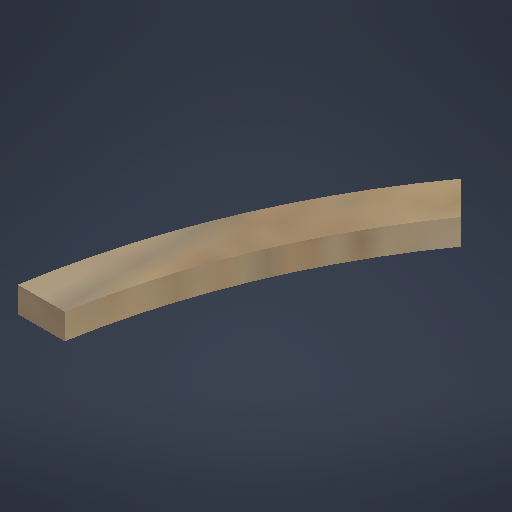
# Autodesk Inventor part: back_upper
Saved by Autodesk Inventor 2026.1 (Build 301233020, 233B)
## iProperties
Created: 2025-09-27
Part Number: back_upper
Material: 木材 (カエデ材)
Document SubType Name: Modeling
Designer: hibik
Density: 0.67 g/cm^3
Appearance: ナチュラル カエデ材 - 光沢 濃い着色
Author: hibik
Autodesk Inventor part; units mm, degrees
ref_plane "YZ Plane" through (0, 0, 0) normal (1, 0, 0) x (0, 1, 0)
ref_plane "XZ Plane" through (0, 0, 0) normal (0, 1, 0) x (-1, 0, 0)
ref_plane "XY Plane" through (0, 0, 0) normal (0, 0, 1) x (1, 0, 0)
sketch "スケッチ1" plane through (0, 0, 0) normal (0, 1, 0) x (-1, 0, 0)
  circle A0 centre (0, 0) radius 178.1675
  circle A1 centre (0, 0) radius 157.8276
  line L0 (168.1877, 0) -> (166.7488, -21.9529)
  line L1 (168.1877, 0) -> (130.1721, 2.4917) construction
  line L2 (249.4344, 0) -> (-249.4344, 0) projected
  line L3 (166.7488, -21.9529) -> (156.7702, -21.2989)
  line L4 (156.7702, -21.2989) -> (158.2091, 0.654) construction
  line L5 (158.2091, 0.654) -> (168.1877, 0)
  line L6 (157.4896, -10.3224) -> (0, 0)
  line L7 (166.7488, -21.9529) -> (162.4568, -43.5302)
  line L8 (162.4568, -43.5302) -> (152.649, -41.5793) construction
  line L9 (152.649, -41.5793) -> (156.9409, -20.002) construction
  line L10 (156.9409, -20.002) -> (166.7488, -21.9529) construction
  line L11 (162.4568, -43.5302) -> (155.3851, -64.3626)
  line L12 (155.3851, -64.3626) -> (145.9158, -61.1482) construction
  line L13 (145.9158, -61.1482) -> (152.9875, -40.3158) construction
  line L14 (152.9875, -40.3158) -> (162.4568, -43.5302) construction
  line L15 (155.3851, -64.3626) -> (145.6548, -84.0938)
  line L16 (145.6548, -84.0938) -> (136.6861, -79.6709) construction
  line L17 (136.6861, -79.6709) -> (146.4164, -59.9397) construction
  line L18 (146.4164, -59.9397) -> (155.3851, -64.3626) construction
  line L19 (0, 0) -> (111.6009, -111.6009)
  line L20 (145.6548, -84.0938) -> (137.3401, -78.5381) construction
  line L21 (137.3401, -78.5381) -> (125.1176, -96.8305) construction
  line L22 (125.1176, -96.8305) -> (133.4323, -102.3862) construction
  line L23 (133.4323, -102.3862) -> (145.6548, -84.0938)
  line L24 (133.4323, -102.3862) -> (125.9139, -95.7927) construction
  line L25 (125.9139, -95.7927) -> (111.4082, -112.3332) construction
  line L26 (111.4082, -112.3332) -> (118.9266, -118.9266)
  line L27 (118.9266, -118.9266) -> (133.4323, -102.3862)
  line L28 (111.6009, -111.6009) -> (118.9266, -118.9266)
  line L29 (166.7488, -21.9529) -> (176.7274, -22.6069) construction
  line L30 (118.9266, -118.9266) -> (125.9834, -125.9834)
  point P0 (154.795, -30.7906)
  point P1 (149.4517, -50.732)
  point P2 (141.5512, -69.8053)
  point P3 (131.2288, -87.6843)
  point P4 (118.661, -104.0629)
  point P5 (157.8276, 0)
  point P6 (178.1675, 0)
  dimension "d0" = 22
  dimension "d1" = 10
  dimension "d2" = 45
  dimension "d4" = 315.6551
  constraints: 60 end point, 11 equal length, 10 parallel, 9 perpendicular, 8 point on circle, 6 midpoint, 3 collinear, 2 centre point, 2 coincident, 1 point on line, 1 tangent
  measures "d0" distance from line of L0.end L1
  measures "d1" distance between parallel lines of L4 L0
  measures "d2" angle of L2 L19
  measures "d4" diameter of A1
extrude "押し出し1" add sketch "スケッチ1" along normal blind 5.5 contours L30 L27 L23 L15 L11 L7 L0 L2 A0 | L28 A1 L2 L0 L7 L11 L15 L23 L27
sketch "スケッチ2" plane through (0, 5.5, 0) normal (0, 1, 0) x (1, 0, 0)
  circle A0 centre (0, 0) radius 309.8276
  line L0 (-168.1877, 0) -> (-166.7488, 21.9529) projected
  line L1 (-166.7488, 21.9529) -> (-162.4568, 43.5302) projected
  line L2 (-162.4568, 43.5302) -> (-155.3851, 64.3626) projected
  line L3 (-155.3851, 64.3626) -> (-145.6548, 84.0938) projected
  line L4 (-133.4323, 102.3862) -> (-145.6548, 84.0938) projected
  line L5 (-118.9266, 118.9266) -> (-133.4323, 102.3862) projected
  line L6 (-167.4682, 10.9764) -> (-166.0294, 32.9293)
  line L7 (-166.0294, 32.9293) -> (-275.7938, 40.1237)
  line L8 (-275.7938, 40.1237) -> (-277.2327, 18.1708)
  line L9 (-277.2327, 18.1708) -> (-167.4682, 10.9764)
  line L10 (-164.6028, 32.7415) -> (-160.3108, 54.3188)
  line L11 (-160.3108, 54.3188) -> (-268.1972, 75.7787)
  line L12 (-268.1972, 75.7787) -> (-272.4892, 54.2015)
  line L13 (-272.4892, 54.2015) -> (-164.6028, 32.7415)
  circle A1 centre (-166.7488, 21.9529) radius 11
  circle A2 centre (-162.4568, 43.5302) radius 11
  line L14 (-158.921, 53.9464) -> (-151.8493, 74.7789)
  line L15 (-151.8493, 74.7789) -> (-256.0116, 110.1372)
  line L16 (-256.0116, 110.1372) -> (-263.0833, 89.3047)
  line L17 (-263.0833, 89.3047) -> (-158.921, 53.9464)
  circle A3 centre (-155.3851, 64.3626) radius 11
  arc A4 (-275.7591, 62.4834) -> (-281.3553, 41.7349) centre (-166.7488, 21.9529) ccw
  line L18 (-178.1663, 0.654) -> (-158.2091, -0.654)
  line L19 (-158.2091, -0.654) -> (-156.7702, 21.2989)
  line L20 (-156.7702, 21.2989) -> (-176.7274, 22.6069)
  line L21 (-176.7274, 22.6069) -> (-178.1663, 0.654)
  line L22 (-177.4468, 11.6305) -> (-275.7938, 40.1237)
  line L23 (-176.7274, 22.6069) -> (-176.008, 33.5834)
  line L24 (-176.008, 33.5834) -> (-275.7591, 62.4834)
  line L25 (-275.7938, 40.1237) -> (-281.3553, 41.7349)
  circle A5 centre (0, 0) radius 137.8276
  line L26 (0, 0) -> (-219.0812, 219.0812)
  line L27 (-111.6009, 111.6009) -> (-125.9834, 125.9834) projected
  line L28 (-433.7586, 0) -> (433.7586, 0) projected
  circle A6 centre (0, 0) radius 279.8276 construction
  arc A7 (-111.6009, 111.6009) -> (-157.8276, 0) centre (0, 0) ccw projected
  point P0 (-158.1662, 0)
  point P1 (-137.8276, 0)
  point P2 (-97.4588, 97.4588)
  point P3 (-309.8276, 0)
  dimension "d7" = 22
  dimension "d10" = 20
  dimension "d11" = 100
  dimension "d12" = 30
  dimension "d14" = 20
  dimension "d17" = 122
  constraints: 42 end point, 9 parallel, 6 centre point, 6 coincident, 6 collinear, 6 midpoint, 5 equal length, 4 perpendicular, 3 point on circle, 2 equal radius, 1 point on line, 1 tangent, 3 other
  measures "d7" distance between parallel lines of L7 L9
  measures "d10" distance between parallel lines of L19 L21
  measures "d11" distance between parallel lines of L23 L8
  measures "d14" radial gap between concentric circles of A5 A7
  measures "d17" radial gap between concentric circles of A7 A6
extrude "押し出し2" add sketch "スケッチ2" against normal blind 5.5 contours L26 L5 L4 L3 A3 L15 L16 L17 A2 L11 L12 L24 A4 L25 L8 L9 L21 L18 L28 A0 | L18 L21 L9 L0 | L0 A1 L19 L28 | A5 L28 A7 A1 A2 A3 L26 | L26 A7 A3 L3 L4 L5 | A1 L21 L20 L0 | L9 L21 A1 | L0 L20 L19 A1 | L19 A7 L28 | L6 A1 L1 | L20 L23 A1 L6 | L1 A1 A7 L19 L20 | L22 L7 L23 A1 L21 | L9 L8 L22 | A1 L23 L21 | A1 A7 L19 | A7 A3 L2 L3 | A3 A7 | A2 L10 L1 | A1 L7 L24 L13 | A2 A7 A1 | L13 L24 L12 L11 A2 | L1 L2 A2 A7 | A1 L23 L7 | L25 A4 L24 L12 L13 L7 | A7 A1 | A7 A2 A3 | L3 L14 A3 | L10 A2 L2 | L13 L12 L24 | A7 A2 | A3 L14 L2 | L17 L16 L15 A3
sketch "スケッチ3" plane through (0, 5.5, 0) normal (0, 1, 0) x (1, 0, 0)
  circle A0 centre (0, 0) radius 157.8276
  arc A1 (-97.4588, 97.4588) -> (-137.8276, 0) centre (0, 0) ccw projected
  line L0 (-97.4588, 97.4588) -> (-219.0812, 219.0812) projected
  line L1 (-309.8276, 0) -> (-137.8276, 0) projected
  arc A2 (-219.0812, 219.0812) -> (-309.8276, 0) centre (0, 0) ccw projected
  point P0 (-157.8276, 0)
  point P1 (-111.6009, 111.6009)
  dimension "d18" = 20
  constraints: 1 centre point, 1 coincident
  measures "d18" radial gap between concentric circles of A0 A1
extrude "押し出し3" cut sketch "スケッチ3" against normal through all contours A0 L1 A2 L0
sketch "スケッチ4" plane through (0, 5.5, 0) normal (0, 1, 0) x (1, 0, 0)
  arc A0 (-111.6009, 111.6009) -> (-157.8276, 0) centre (0, 0) ccw projected
  line L0 (-157.8276, 0) -> (-137.8276, 0)
  line L1 (-137.8276, 0) -> (-137.8276, 25)
  line L2 (-137.8276, 25) -> (-157.8276, 25)
  line L3 (-157.8276, 25) -> (-157.8276, 0)
  arc A1 (-97.4588, 97.4588) -> (-137.8276, 0) centre (0, 0) ccw projected
  line L4 (-97.4588, 97.4588) -> (-111.6009, 111.6009)
  line L5 (-111.6009, 111.6009) -> (-129.2786, 93.9233)
  line L6 (-129.2786, 93.9233) -> (-115.1365, 79.7811)
  line L7 (-115.1365, 79.7811) -> (-97.4588, 97.4588)
  dimension "d21" = 25
  dimension "d22" = 25
  constraints: 16 end point, 4 parallel, 2 perpendicular, 1 horizontal
  measures "d21" distance of L0.end L1.end
  measures "d22" distance between parallel lines of L4 L6
extrude "押し出し4" cut sketch "スケッチ4" against normal through all contours L4 L7 L6 A0 | A0 L6 L5 | L2 L1 L0 A0 | A0 L3 L2
fillet "フィレット1" radius 1 2 edges at (-97.4588, 2.75, -97.4588) (-137.8276, 2.75, 0)
sketch "スケッチ5" plane through (0, 5.5, 0) normal (0, 1, 0) x (1, 0, 0)
  circle A0 centre (0, 0) radius 147.8276
  arc A1 (-127.8696, 92.5143) -> (-155.835, 25) centre (0, 0) ccw projected
  arc A2 (-137.8276, 23.48) -> (-135.842, 23.3109) centre (-136.8276, 23.48) ccw projected
  arc A3 (-112.5381, 79.5715) -> (-135.842, 23.3109) centre (0, 0) ccw projected
  arc A4 (-112.5381, 79.5715) -> (-114.0617, 80.8559) centre (-113.3546, 80.1488) ccw projected
  line L0 (-114.0617, 80.8559) -> (-115.1365, 79.7811) projected
  line L1 (-115.1365, 79.7811) -> (-127.8696, 92.5143) projected
  arc A5 (-127.8696, 92.5143) -> (-155.835, 25) centre (0, 0) ccw projected
  line L2 (-155.835, 25) -> (-137.8276, 25) projected
  line L3 (-137.8276, 25) -> (-137.8276, 23.48) projected
  point P0 (-120.7019, 85.3466)
  point P1 (-145.6983, 25)
  dimension "d26" = 10
  constraints: 1 centre point, 1 coincident
  measures "d26" radial gap between concentric circles of A1 A0
extrude "押し出し5" cut sketch "スケッチ5" against normal through all contours L1 L0 A4 A3 A2 L3 L2 A0 picked at (-137.0003, 45.2919)
equation "\"d22\" = d21"
